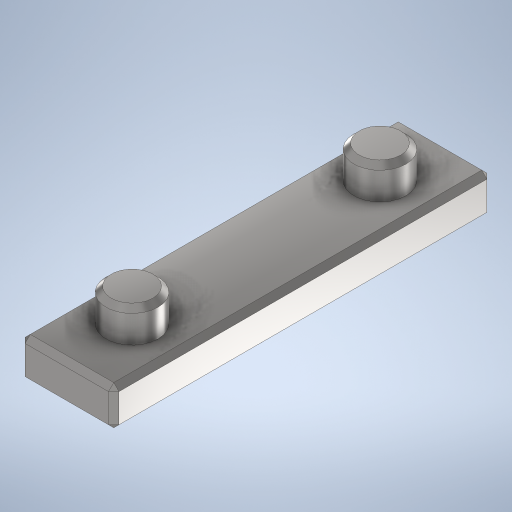
# Autodesk Inventor part: hydraulic_mech
Saved by Autodesk Inventor 2023 (Build 270158000, 158)
## iProperties
Created: 2023-11-19
Part Number: hydraulic_mech
Material: Steel, Mild
Document SubType Name: Modeling
Designer: Beatrice
Density: 7.85 g/cm^3
Appearance: Semi-Polished
Author: Beatrice
Autodesk Inventor part; units mm, degrees
ref_plane "YZ Plane" through (0, 0, 0) normal (1, 0, 0) x (0, 1, 0)
ref_plane "XZ Plane" through (0, 0, 0) normal (0, 1, 0) x (-1, 0, 0)
ref_plane "XY Plane" through (0, 0, 0) normal (0, 0, 1) x (1, 0, 0)
sketch "Sketch1" plane through (0, 0, 0) normal (0, 0, 1) x (1, 0, 0)
  line L0 (223.4483, -72.5) -> (-46.5517, -72.5)
  line L1 (-46.5517, -72.5) -> (-46.5517, 72.5)
  line L2 (-46.5517, 72.5) -> (223.4483, 72.5)
  line L3 (223.4483, 72.5) -> (223.4483, -72.5)
  line L4 (223.4483, -72.5) -> (-46.5517, 72.5) construction
  line L5 (-46.5517, -72.5) -> (223.4483, 72.5) construction
  circle A0 centre (0, 47.5) radius 10
  line L6 (18, -72.5) -> (-18, -72.5)
  line L7 (-18, -72.5) -> (-18, 72.5)
  line L8 (-18, 72.5) -> (18, 72.5)
  line L9 (18, 72.5) -> (18, -72.5)
  line L10 (18, -72.5) -> (-18, 72.5) construction
  line L11 (-18, -72.5) -> (18, 72.5) construction
  line L12 (-100.5517, 0) -> (277.4483, 0) construction
  line L13 (0, 101.5) -> (0, -101.5) construction
  circle A1 centre (0, -47.5) radius 10
  line L14 (0, -101.5) -> (0, 101.5) construction
  circle A2 centre (0, 0) radius 15
  point P0 (88.4483, 0)
  dimension "d0" = 145
  dimension "d1" = 270
  dimension "d2" = 20
  dimension "d3" = 25
  dimension "d4" = 36
  dimension "d5" = 30
  constraints: 26 end point, 4 midpoint, 4 parallel, 3 centre point, 3 symmetric about line, 2 horizontal, 2 perpendicular, 2 point on line, 1 coincident, 1 horizontal alignment, 1 vertical alignment, 1 other
  measures "d0" distance of L0.end L1.end
  measures "d1" distance of L0.start L0.end
  measures "d2" diameter of A0
  measures "d3" distance from line of L2 A0.centre
  measures "d4" distance between parallel lines of L9 L7
  measures "d5" diameter of A2
extrude "Extrusion1" add sketch "Sketch1" along normal mid plane 15 contours L0 L7 L2 L9
extrude "Extrusion2" add sketch "Sketch1" against normal blind 7.5 contours A0 | A1
extrude "Extrusion3" add sketch "Sketch1" along normal blind 20 contours A0 | A1
sketch "Sketch2" plane through (0, 0, 7.5) normal (0, 0, 1) x (1, 0, 0)
  line L0 (18, 72.5) -> (-18, 72.5) projected
  line L1 (-18, 72.5) -> (-18, -72.5) projected
  line L2 (-18, -72.5) -> (18, -72.5) projected
  line L3 (18, -72.5) -> (18, 72.5) projected
  circle A0 centre (0, 0) radius 15 projected
  circle A1 centre (0, -47.5) radius 10 projected
  circle A2 centre (0, 47.5) radius 10 projected
extrude "Extrusion4" add sketch "Sketch2" against normal blind 6 contours A0
chamfer "Chamfer1" distance 2 angle 45 13 edges at (0, -72.5, 7.5) (18, -72.5, 0) (0, -72.5, -7.5) (18, 0, -7.5) (18, 0, 7.5) (18, 72.5, 0) (0, 72.5, 7.5) (-18, 0, 7.5) (-10, 47.5, 20) (-10, -47.5, 20) (-18, 0, -7.5) (-18, -72.5, 0) (-18, 72.5, 0)
body "Solid1"
